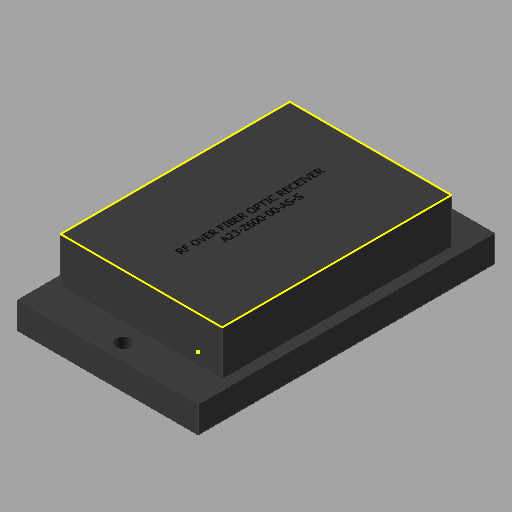
# Autodesk Inventor part: receiver box
Saved by Autodesk Inventor 2025.3 (Build 293356000, 356)
## iProperties
Created: 2025-10-16
Part Number: receiver box
Material: Generic
Document SubType Name: Modeling
Designer: sonata
Density: 1 g/cm^3
Appearance: Default
Author: sonata
Autodesk Inventor part; units mm, degrees
ref_plane "YZ Plane" through (0, 0, 0) normal (1, 0, 0) x (0, 1, 0)
ref_plane "XZ Plane" through (0, 0, 0) normal (0, 1, 0) x (-1, 0, 0)
ref_plane "XY Plane" through (0, 0, 0) normal (0, 0, 1) x (1, 0, 0)
sketch "Sketch1" plane through (0, 0, 0) normal (0, 1, 0) x (-1, 0, 0)
  line L0 (0, 0) -> (78.0034, 0)
  line L1 (78.0034, 0) -> (78.0034, -127.9906)
  line L2 (78.0034, -127.9906) -> (0, -127.9906)
  line L3 (0, -127.9906) -> (0, 0)
  dimension "d0" = 127.9906
  dimension "d1" = 78.0034
  constraints: 8 end point, 2 parallel, 1 horizontal, 1 perpendicular
  measures "d0" distance of L0.end L1.end
  measures "d1" distance of L0.start L0.end
extrude "Extrusion1" add sketch "Sketch1" along normal blind 11.5062
sketch "Sketch2" plane through (0, 11.5062, 0) normal (0, 1, 0) x (1, 0, 0)
  line L0 (-78.0034, 0) -> (0, 0) projected
  line L1 (0, 127.9906) -> (-78.0034, 127.9906) projected
  line L2 (-39.0017, 0) -> (-39.0017, 127.9906) construction
  line L3 (-78.0034, 127.9906) -> (-78.0034, 0) construction
  line L4 (-78.0034, 63.9953) -> (0, 63.9953) construction
  line L5 (0, 0) -> (0, 127.9906) construction
  point P0 (-39.0017, 6.9977)
  point P1 (-39.0017, 120.9929)
  dimension "d4" = 113.9952
  dimension "d5" = 56.9976
  constraints: 4 end point, 4 midpoint, 2 point on line
  measures "d4" distance of point (-39.002, 120.993) point (-39.002, 6.998)
  measures "d5" distance from line of L4 point (-39.002, 6.998)
hole "Hole1" at (-39.0017, 11.5062, -6.9977) at (-39.0017, 11.5062, -120.9929) direction (0, -1, 0) diameter 3.9878 depth 11.5062 counterbore diameter 7.112 counterbore depth 7.0612
sketch "Sketch3" plane through (0, 11.5062, 0) normal (0, 1, 0) x (1, 0, 0)
  line L0 (-73.9267, 14.4653) -> (-4.0767, 14.4653)
  line L1 (-4.0767, 14.4653) -> (-4.0767, 113.5253)
  line L2 (-4.0767, 113.5253) -> (-73.9267, 113.5253)
  line L3 (-73.9267, 113.5253) -> (-73.9267, 14.4653)
  line L4 (-78.0034, 0) -> (0, 0) projected
  line L5 (0, 0) -> (0, 127.9906) projected
  line L6 (0, 63.9953) -> (-78.0034, 63.9953) construction
  line L7 (-78.0034, 127.9906) -> (-78.0034, 0) projected
  line L8 (-39.0017, 0) -> (-39.0017, 127.9906) construction
  line L9 (0, 127.9906) -> (-78.0034, 127.9906) projected
  point P0 (-39.0017, 63.9953)
  dimension "d13" = 99.06
  dimension "d15" = 69.85
  dimension "d16" = 49.53
  dimension "d17" = 34.925
  constraints: 12 end point, 6 midpoint, 2 parallel, 1 horizontal, 1 perpendicular
  measures "d13" distance between parallel lines of L2 L0
  measures "d15" distance between parallel lines of L1 L3
  measures "d16" distance between parallel lines of L6 L0
  measures "d17" distance between parallel lines of L8 L1
extrude "Extrusion2" add sketch "Sketch3" along normal blind 30.988 from surface at -11.5062 contours L3 L2 L1 L0
sketch "Sketch4" plane through (-73.9267, 30.988, -14.4653) normal (0, 1, 0) x (1, 0, 0)
  line L0 (30.8017, -0.4384) -> (30.8017, 99.4984) construction
  line L1 (30.8017, 99.4984) -> (42.6663, 99.4984) construction
  line L2 (42.6663, 99.4984) -> (42.6663, -0.4384) construction
  line L3 (42.6663, -0.4384) -> (30.8017, -0.4384) construction
  line L4 (69.85, 0) -> (0, 0) projected
  line L5 (0, 99.06) -> (69.85, 99.06) projected
  line L6 (0, 0) -> (0, 99.06) projected
  line L7 (69.85, 99.06) -> (69.85, 0) projected
  point P0 (73.9267, -14.4653)
  constraints: 2 other
body "Solid1"
